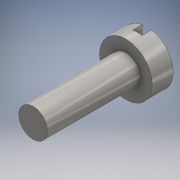
# Autodesk Inventor part: screw12x3mm
Saved by Autodesk Inventor 2016 (Build 200138000, 138)
## iProperties
Created: 2016-06-04
Part Number: screw12x3mm
Material: Stainless Steel
Document SubType Name: Modeling
Designer: hesaon
Density: 8 g/cm^3
Appearance: Semi-Polished
Author: hesaon
Autodesk Inventor part; units mm, degrees
ref_plane "YZ Plane" through (0, 0, 0) normal (1, 0, 0) x (0, 1, 0)
ref_plane "XZ Plane" through (0, 0, 0) normal (0, 1, 0) x (-1, 0, 0)
ref_plane "XY Plane" through (0, 0, 0) normal (0, 0, 1) x (1, 0, 0)
sketch "Sketch1" plane through (0, 0, 0) normal (0, 1, 0) x (-1, 0, 0)
  circle A0 centre (0, 0) radius 1.5
  dimension "d0" = 3
  constraints: 1 centre point, 1 coincident
  measures "d0" diameter of A0
extrude "Extrusion1" add sketch "Sketch1" along normal blind 9.7
sketch "Sketch2" plane through (0, 9.7, 0) normal (0, 1, 0) x (1, 0, 0)
  circle A0 centre (0, 0) radius 2.75
  dimension "d3" = 5.5
  constraints: 1 centre point, 1 coincident
  measures "d3" diameter of A0
extrude "Extrusion2" add sketch "Sketch2" along normal blind 2.2
sketch "Sketch3" plane through (0, 11.9, 0) normal (0, 1, 0) x (1, 0, 0)
  line L0 (0.5, -4.7072) -> (-0.5, -4.7072)
  line L1 (-0.5, -4.7072) -> (-0.5, 4.7072)
  line L2 (-0.5, 4.7072) -> (0.5, 4.7072)
  line L3 (0.5, 4.7072) -> (0.5, -4.7072)
  line L4 (0.5, -4.7072) -> (-0.5, 4.7072) construction
  line L5 (-0.5, -4.7072) -> (0.5, 4.7072) construction
  point P0 (0, 0)
  dimension "d6" = 1
  constraints: 12 end point, 2 midpoint, 2 parallel, 1 horizontal, 1 perpendicular
  measures "d6" distance of L1.end L2.end
extrude "Extrusion3" cut sketch "Sketch3" against normal blind 1
body "Solid1"
